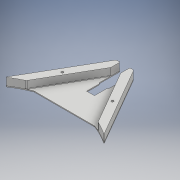
# Autodesk Inventor part: Delta motor covers
Saved by Autodesk Inventor 2018 (Build 220112000, 112)
## iProperties
Created: 2018-02-11
Part Number: Delta motor covers
Material: Generic
Document SubType Name: Modeling
Designer: elect
Density: 1 g/cm^3
Appearance: Default
Author: elect
Autodesk Inventor part; units mm, degrees
ref_plane "YZ Plane" through (0, 0, 0) normal (1, 0, 0) x (0, 1, 0)
ref_plane "XZ Plane" through (0, 0, 0) normal (0, 1, 0) x (-1, 0, 0)
ref_plane "XY Plane" through (0, 0, 0) normal (0, 0, 1) x (1, 0, 0)
sketch "Sketch1" plane through (0, 0, 0) normal (0, 0, 1) x (1, 0, 0)
  line L0 (-0.0006, 0.0163) -> (155.9994, 0.0163) construction
  line L1 (-0.0006, 0.0163) -> (186.9994, 0.0163) construction
  line L2 (-0.001, 176.3023) -> (65.3232, 176.3024)
  line L3 (-0.001, 176.3023) -> (-65.3251, 176.3022)
  line L4 (-0.0011, 232.6453) -> (-8.5011, 232.6453)
  line L5 (-0.0011, 232.6453) -> (8.4989, 232.6453)
  line L6 (8.4989, 232.6453) -> (8.4989, 259.6453)
  line L7 (8.4989, 259.6453) -> (10.6202, 261.7666)
  line L8 (10.6202, 261.7666) -> (10.6202, 307.0166)
  line L9 (-8.5011, 232.6453) -> (-8.5011, 259.6453)
  line L10 (-8.5011, 259.6453) -> (-10.6224, 261.7666)
  line L11 (-10.6224, 261.7666) -> (-10.6224, 307.0166)
  arc A0 (-65.3251, 176.3022) -> (-106.8225, 154.7195) centre (-0.0006, 0.0163) ccw
  line L12 (106.8278, 154.715) -> (18.9007, 307.0166)
  arc A1 (106.8278, 154.715) -> (65.3232, 176.3024) centre (-0.0006, 0.0163) ccw
  line L13 (-106.8225, 154.7195) -> (-18.8764, 307.0166)
  line L14 (-17.2883, 309.7666) -> (-17.2389, 309.8522)
  line L15 (17.3131, 309.7666) -> (17.2572, 309.8635)
  line L16 (-10.6224, 307.0166) -> (-18.8764, 307.0166)
  line L17 (10.6202, 307.0166) -> (18.9007, 307.0166)
  point P0 (0, 0)
  point P1 (-0.0006, 0.0163)
  dimension "d48" = 175.8662
  dimension "d49" = 8.2539
  constraints: 36 end point, 4 point on circle, 3 horizontal, 2 centre point, 2 coincident, 2 parallel, 2 point on line, 2 vertical
  measures "d48" distance of L13.start L13.end
  measures "d49" distance of L11.end L13.end
extrude "Extrusion1" add sketch "Sketch1" along normal blind 2
sketch "Sketch2" plane through (0, 0, 2) normal (0, 0, 1) x (1, 0, 0)
  line L0 (0, 0) -> (188, 0) construction
  line L1 (-106.8086, 154.7124) -> (-18.8656, 307.0341)
  line L2 (-18.8656, 307.0341) -> (-10.6116, 307.0341)
  line L3 (-10.6116, 307.0341) -> (-10.6116, 287.3305)
  line L4 (-77.6515, 171.214) -> (-10.6116, 287.3305)
  line L5 (-31.2071, 251.6581) -> (-77.6515, 171.214)
  line L6 (106.8086, 154.7124) -> (18.8656, 307.0341)
  line L7 (18.8656, 307.0341) -> (10.6116, 307.0341)
  line L8 (10.6116, 307.0341) -> (10.6116, 287.3301)
  line L9 (10.6116, 287.3301) -> (77.6512, 171.2142)
  arc A0 (-77.6515, 171.214) -> (-106.8086, 154.7124) centre (0, 0) ccw
  arc A1 (106.8086, 154.7124) -> (77.6512, 171.2142) centre (0, 0) ccw
  dimension "d50" = 175.886
  dimension "d52" = 8.254
  dimension "d56" = 19.7036
  dimension "d58" = 8.254
  dimension "d59" = 19.704
  dimension "d60" = 150
  constraints: 20 end point, 4 point on circle, 3 horizontal, 2 centre point, 1 coincident, 1 perpendicular, 1 point on line, 1 vertical
  measures "d50" distance of L1.start L1.end
  measures "d52" distance of L1.end L2.end
  measures "d56" distance of L2.end L3.end
  measures "d58" distance of L6.end L7.end
  measures "d59" distance of L7.end L8.end
  measures "d60" angle of L9 L8
extrude "Extrusion2" add sketch "Sketch2" along normal blind 16
sketch "Sketch3" plane through (0, 0, 0) normal (0, 0, -1) x (-1, 0, 0)
  circle A0 centre (0, 0) radius 188
  line L0 (0, 0) -> (-106.8086, 154.7124)
  line L1 (0, 0) -> (188, 0) construction
  line L2 (0, 0) -> (106.8086, 154.7124)
  line L3 (-106.8086, 154.7124) -> (-18.8656, 307.0341)
  line L4 (-106.8086, 154.7124) -> (69.0774, 154.7124) construction
  line L5 (-18.8656, 307.0341) -> (-10.2054, 302.0341)
  line L6 (-10.2054, 302.0341) -> (-54.1769, 225.8732)
  line L7 (106.8086, 154.7124) -> (18.8656, 307.0341)
  line L8 (106.8086, 154.7124) -> (282.6946, 154.7124) construction
  line L9 (18.8656, 307.0341) -> (10.2054, 302.0341)
  line L10 (10.2054, 302.0341) -> (54.1769, 225.8732)
  dimension "d63" = 376
  dimension "d64" = 124.62
  dimension "d65" = 175.886
  dimension "d66" = 60
  dimension "d67" = 10
  dimension "d68" = 87.943
  dimension "d69" = 120
  constraints: 22 end point, 4 perpendicular, 3 equal length, 3 horizontal, 2 point on circle, 1 centre point, 1 coincident
  measures "d63" diameter of A0
  measures "d64" angle of L1 L0
  measures "d65" distance of L0.end L3.end
  measures "d66" angle of L4 L3
  measures "d67" distance of L3.end L5.end
  measures "d68" distance of L5.end L6.end
  measures "d69" angle of L8 L7
hole "Hole1" at (54.1769, 225.8732, 0) at (-54.1769, 225.8732, 0) direction (0, 0, 1) diameter 5 depth 18 tip angle 118 counterbore diameter 10 counterbore depth 13
fillet "Fillet1" radius 5 1 edges at (-18.8656, 307.0341, 10)
fillet "Fillet2" radius 5 1 edges at (-18.8764, 307.0166, 1)
fillet "Fillet3" radius 2 1 edges at (-10.6116, 307.0341, 10)
fillet "Fillet4" radius 5 2 edges at (18.8656, 307.0341, 10) (18.9007, 307.0166, 1)
fillet "Fillet5" radius 2 1 edges at (10.6116, 307.0341, 10)
fillet "Fillet6" radius 5 1 edges at (77.6512, 171.2142, 10)
fillet "Fillet7" radius 5 1 edges at (-77.6515, 171.214, 10)
fillet "Fillet8" radius 0.5 1 edges at (106.8086, 154.7124, 10)
fillet "Fillet9" radius 0.5 1 edges at (106.8278, 154.715, 1)
fillet "Fillet10" radius 0.5 2 edges at (-106.8086, 154.7124, 10) (-106.8225, 154.7195, 1)
fillet "Fillet11" radius 1 2 edges at (43.7372, 229.9549, 2) (77.6739, 171.5341, 2)
fillet "Fillet12" radius 1 2 edges at (-43.7385, 229.9531, 2) (-77.6719, 171.5363, 2)
body "Solid1"
